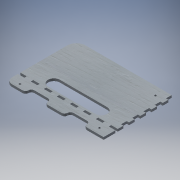
# Autodesk Inventor part: LatoPy
Saved by Autodesk Inventor 2018.3 (Build 223284000, 284)
## iProperties
Created: 2019-03-05
Part Number: LatoPy
Material: Generico
Document SubType Name: Modeling
Designer: AlfyPc
Density: 1 g/cm^3
Appearance: Legno - Verniciato - Bianco
Author: AlfyPc
Autodesk Inventor part; units mm, degrees
(part 1 of 3)
ref_plane "YZ Plane" through (0, 0, 0) normal (1, 0, 0) x (0, 1, 0)
ref_plane "XZ Plane" through (0, 0, 0) normal (0, 1, 0) x (-1, 0, 0)
ref_plane "XY Plane" through (0, 0, 0) normal (0, 0, 1) x (1, 0, 0)
sketch "Schizzo1" plane through (0, 0, 0) normal (0, 0, 1) x (1, 0, 0)
  line L0 (4, 17) -> (0, 17) construction
  line L1 (0, 17) -> (0, 95) construction
  line L2 (0, 95) -> (4, 95) construction
  line L3 (4, 95) -> (4, 17) construction
  line L4 (4, -4) -> (4, -24) construction
  line L5 (4, -24) -> (0, -24) construction
  line L6 (0, -24) -> (0, -4) construction
  line L7 (0, 0) -> (0, 11) construction
  line L8 (0, 11) -> (4, 11) construction
  line L9 (4, 11) -> (4, 0) construction
  line L10 (-161, -24) -> (-161, 95)
  line L11 (-161, 95) -> (4, 95)
  line L12 (4, 95) -> (4, -24)
  line L13 (-133, -24) -> (-161, -24)
  arc A0 (-133, -24) -> (-128, -19) centre (-133, -19) ccw
  arc A1 (-123, -14) -> (-128, -19) centre (-123, -19) ccw
  line L14 (-100, -14) -> (-123, -14)
  arc A2 (-95, -19) -> (-100, -14) centre (-100, -19) ccw
  arc A3 (-95, -19) -> (-90, -24) centre (-90, -19) ccw
  line L15 (-67, -24) -> (-90, -24)
  arc A4 (-67, -24) -> (-62, -19) centre (-67, -19) ccw
  arc A5 (-57, -14) -> (-62, -19) centre (-57, -19) ccw
  line L16 (-34, -14) -> (-57, -14)
  arc A6 (-29, -19) -> (-34, -14) centre (-34, -19) ccw
  arc A7 (-29, -19) -> (-24, -24) centre (-24, -19) ccw
  line L17 (4, -24) -> (-24, -24)
  line L18 (-117, 13) -> (-37, 13) construction
  line L19 (-117, 3) -> (-37, 3)
  line L20 (-37, 23) -> (-117, 23)
  arc A8 (-117, 23) -> (-117, 3) centre (-117, 13) ccw
  arc A9 (-37, 3) -> (-37, 23) centre (-37, 13) ccw
  line L21 (-161, -4) -> (-150, -4) projected
  line L22 (-150, 0) -> (-150, -4) projected
  line L23 (-139, -4) -> (-128, -4) projected
  line L24 (-128, 0) -> (-128, -4) projected
  line L25 (-139, 0) -> (-128, 0) projected
  line L26 (-139, 0) -> (-139, -4) projected
  line L27 (-117, -4) -> (-106, -4) projected
  line L28 (-106, 0) -> (-106, -4) projected
  line L29 (-117, 0) -> (-106, 0) projected
  line L30 (-117, 0) -> (-117, -4) projected
  line L31 (-95, -4) -> (-84, -4) projected
  line L32 (-84, 0) -> (-84, -4) projected
  line L33 (-95, 0) -> (-84, 0) projected
  line L34 (-95, 0) -> (-95, -4) projected
  line L35 (-73, -4) -> (-62, -4) projected
  line L36 (-62, 0) -> (-62, -4) projected
  line L37 (-73, 0) -> (-62, 0) projected
  line L38 (-73, 0) -> (-73, -4) projected
  line L39 (-51, -4) -> (-40, -4) projected
  line L40 (-40, 0) -> (-40, -4) projected
  line L41 (-51, 0) -> (-40, 0) projected
  line L42 (-51, 0) -> (-51, -4) projected
  line L43 (-29, -4) -> (-18, -4) projected
  line L44 (-18, 0) -> (-18, -4) projected
  line L45 (-29, 0) -> (-18, 0) projected
  line L46 (-29, 0) -> (-29, -4) projected
  line L47 (-7, -4) -> (4, -4) projected
  line L48 (4, 0) -> (4, -4) projected
  line L49 (-7, 0) -> (4, 0) projected
  line L50 (-7, 0) -> (-7, -4) projected
  line L51 (-161, 0) -> (-150, 0) projected
  line L52 (-161, 0) -> (-161, -4) projected
  point P0 (-77, 13)
  dimension "d0" = 80
  constraints: 44 end point, 20 point on circle, 10 centre point, 6 vertical, 4 horizontal, 4 tangent, 2 parallel, 1 midpoint, 10 other
  measures "d0" distance of L18.start L18.end
extrude "Estrusione1" add sketch "Schizzo1" along normal blind 4 contours L10 L21 L22 L51 L11 L12 L49 L50 L47 L17 A7 A6 L16 A5 A4 L15 A3 A2 L14 A1 A0 L13
sketch "Schizzo2" plane through (0, 0, 4) normal (0, 0, 1) x (1, 0, 0)
  line L0 (0, 76) -> (4, 76)
  line L1 (4, 76) -> (4, 66.5)
  line L2 (4, 66.5) -> (0, 66.5)
  line L3 (0, 66.5) -> (0, 76)
  line L4 (4, 85.5) -> (0, 85.5)
  line L5 (0, 85.5) -> (0, 95)
  line L6 (0, 95) -> (4, 95)
  line L7 (4, 95) -> (4, 85.5)
  line L8 (0, 38) -> (4, 38)
  line L9 (4, 38) -> (4, 28.5)
  line L10 (4, 28.5) -> (0, 28.5)
  line L11 (0, 28.5) -> (0, 38)
  line L12 (4, 47.5) -> (0, 47.5)
  line L13 (0, 47.5) -> (0, 57)
  line L14 (0, 57) -> (4, 57)
  line L15 (4, 57) -> (4, 47.5)
  line L16 (4, 9.5) -> (0, 9.5)
  line L17 (0, 9.5) -> (0, 19)
  line L18 (0, 19) -> (4, 19)
  line L19 (4, 19) -> (4, 9.5)
  point P0 (0, 0)
  constraints: 40 end point, 10 horizontal, 10 vertical, 20 other
extrude "Estrusione2" cut sketch "Schizzo2" against normal blind 4
fillet "Raccordo1" radius 15 1 edges at (-161, 95, 2)
fillet "Raccordo2" radius 10 1 edges at (-161, -24, 2)
sketch "Schizzo3" plane through (0, 0, 4) normal (0, 0, 1) x (1, 0, 0)
  line L0 (-146.15, 0) -> (-142.85, 0) projected
  line L1 (-14.15, 0) -> (-10.85, 0) projected
  line L2 (-144.5, 0) -> (-144.5, -17) construction
  circle A0 centre (-144.5, -17) radius 1.65
  line L3 (0, 79.1) -> (0, 82.4) construction
  line L4 (0, -15.65) -> (0, -12.35) construction
  line L5 (0, -14) -> (-13, -14) construction
  line L6 (0, 80.75) -> (-13, 80.75) construction
  circle A1 centre (-13, 80.75) radius 1.65
  circle A2 centre (-13, -14) radius 1.65
  point P0 (0, 0)
  dimension "d8" = 3.3
  dimension "d13" = 13
  dimension "d14" = 13
  dimension "d15" = 3.3
  dimension "d16" = 3.3
  dimension "d17" = 17
  constraints: 6 end point, 3 centre point, 3 coincident, 3 midpoint, 2 horizontal, 1 vertical
  measures "d8" diameter of A0
  measures "d13" distance of L5.start L5.end
  measures "d14" distance of L6.start L6.end
  measures "d15" diameter of A1
  measures "d16" diameter of A2
  measures "d17" distance of L2.start L2.end
extrude "Estrusione3" cut sketch "Schizzo3" against normal blind 4
sketch "Schizzo4" plane through (0, 0, 0) normal (0, 0, -1) x (-1, 0, 0)
  line L0 (22.8203, 78.8425) -> (60.2555, 78.8425)
  line L1 (60.2555, 78.8425) -> (60.2555, 30)
  line L2 (60.2555, 30) -> (22.8203, 30)
  line L3 (22.8203, 30) -> (22.8203, 78.8425)
  line L4 (68.3569, 29.9673) -> (68.3569, 80.7398) construction
  line L5 (68.3569, 80.7398) -> (122.609, 80.7398) construction
  line L6 (122.609, 80.7398) -> (122.609, 29.9673) construction
  line L7 (122.609, 29.9673) -> (68.3569, 29.9673) construction
  spline S0 degree 2 poles (71.5343, 79.079) (71.5343, 78.615) (71.1438, 77.902) (70.4223, 77.5144) (69.9498, 77.5144) knots 0 0 0 1 2 3 3 3
  line L8 (69.9498, 77.5144) -> (68.6568, 77.5144)
  line L9 (68.6568, 77.5144) -> (68.6568, 80.5644)
  line L10 (68.6568, 80.5644) -> (69.9215, 80.5644)
  spline S1 degree 2 poles (69.9215, 80.5644) (71.5343, 80.5644) (71.5343, 79.079) knots 0 0 0 1 1 1
  spline S2 degree 2 poles (70.5581, 79.0705) (70.5581, 79.2912) (70.3771, 79.6505) (70.0404, 79.8457) (69.814, 79.8457) knots 0 0 0 1 2 3 3 3
  line L11 (69.814, 79.8457) -> (69.5764, 79.8457)
  line L12 (69.5764, 79.8457) -> (69.5764, 78.233)
  line L13 (69.5764, 78.233) -> (69.8338, 78.233)
  spline S3 degree 2 poles (69.8338, 78.233) (70.1649, 78.233) (70.5581, 78.6857) (70.5581, 79.0705) knots 0 0 0 1 2 2 2
  spline S4 degree 2 poles (72.6632, 78.3462) (72.6858, 78.2047) (72.9631, 78.0463) (73.1894, 78.0463) knots 0 0 0 1 2 2 2
  spline S5 degree 2 poles (73.1894, 78.0463) (73.5063, 78.0463) (73.7892, 78.1679) knots 0 0 0 1 1 1
  line L14 (73.7892, 78.1679) -> (73.7892, 77.5936)
  spline S6 degree 2 poles (73.7892, 77.5936) (73.461, 77.4606) (72.9885, 77.4606) knots 0 0 0 1 1 1
  spline S7 degree 2 poles (72.9885, 77.4606) (72.4198, 77.4606) (71.7861, 78.0435) (71.7861, 78.5556) knots 0 0 0 1 2 2 2
  spline S8 degree 2 poles (71.7861, 78.5556) (71.7861, 78.9064) (72.0633, 79.4411) (72.6094, 79.7467) (72.9404, 79.7467) knots 0 0 0 1 2 3 3 3
  spline S9 degree 2 poles (72.9404, 79.7467) (73.2771, 79.7467) (73.7581, 79.4836) (74.0071, 79.0054) (74.0071, 78.6857) knots 0 0 0 1 2 3 3 3
  line L15 (74.0071, 78.6857) -> (74.0071, 78.3462)
  line L16 (74.0071, 78.3462) -> (72.6632, 78.3462)
  spline S10 degree 2 poles (73.2064, 78.8215) (73.2064, 79.1978) (72.9376, 79.1978) knots 0 0 0 1 1 1
  spline S11 degree 2 poles (72.9376, 79.1978) (72.8244, 79.1978) (72.6716, 78.9913) (72.6575, 78.8215) knots 0 0 0 1 2 2 2
  line L17 (72.6575, 78.8215) -> (73.2064, 78.8215)
  line L18 (75.9055, 77.5144) -> (74.8304, 77.5144)
  line L19 (74.8304, 77.5144) -> (74.1033, 79.6929)
  line L20 (74.1033, 79.6929) -> (75.0483, 79.6929)
  line L21 (75.0483, 79.6929) -> (75.3142, 78.5046)
  spline S12 degree 2 poles (75.3142, 78.5046) (75.3765, 78.216) (75.385, 78.0718) knots 0 0 0 1 1 1
  line L22 (75.385, 78.0718) -> (75.3963, 78.0718)
  spline S13 degree 2 poles (75.3963, 78.0718) (75.4019, 78.1142) (75.4161, 78.2047) (75.7245, 79.6929) knots 0 0 0 1 2 2 2
  line L23 (75.7245, 79.6929) -> (76.6638, 79.6929)
  line L24 (76.6638, 79.6929) -> (75.9055, 77.5144)
  spline S14 degree 2 poles (77.6625, 78.3462) (77.6852, 78.2047) (77.9625, 78.0463) (78.1888, 78.0463) knots 0 0 0 1 2 2 2
  spline S15 degree 2 poles (78.1888, 78.0463) (78.5057, 78.0463) (78.7886, 78.1679) knots 0 0 0 1 1 1
  line L25 (78.7886, 78.1679) -> (78.7886, 77.5936)
  spline S16 degree 2 poles (78.7886, 77.5936) (78.4604, 77.4606) (77.9879, 77.4606) knots 0 0 0 1 1 1
  spline S17 degree 2 poles (77.9879, 77.4606) (77.4192, 77.4606) (76.7855, 78.0435) (76.7855, 78.5556) knots 0 0 0 1 2 2 2
  spline S18 degree 2 poles (76.7855, 78.5556) (76.7855, 78.9064) (77.0627, 79.4411) (77.6088, 79.7467) (77.9398, 79.7467) knots 0 0 0 1 2 3 3 3
  spline S19 degree 2 poles (77.9398, 79.7467) (78.2765, 79.7467) (78.7575, 79.4836) (79.0065, 79.0054) (79.0065, 78.6857) knots 0 0 0 1 2 3 3 3
  line L26 (79.0065, 78.6857) -> (79.0065, 78.3462)
  line L27 (79.0065, 78.3462) -> (77.6625, 78.3462)
  spline S20 degree 2 poles (78.2058, 78.8215) (78.2058, 79.1978) (77.937, 79.1978) knots 0 0 0 1 1 1
  spline S21 degree 2 poles (77.937, 79.1978) (77.8238, 79.1978) (77.671, 78.9913) (77.6569, 78.8215) knots 0 0 0 1 2 2 2
  line L28 (77.6569, 78.8215) -> (78.2058, 78.8215)
  line L29 (79.3205, 77.5144) -> (79.3205, 80.7398)
  line L30 (79.3205, 80.7398) -> (80.2259, 80.7398)
  line L31 (80.2259, 80.7398) -> (80.2259, 77.5144)
  line L32 (80.2259, 77.5144) -> (79.3205, 77.5144)
  spline S22 degree 2 poles (83.0835, 78.6433) (83.0835, 78.0916) (82.4186, 77.4606) (81.8216, 77.4606) knots 0 0 0 1 2 2 2
  spline S23 degree 2 poles (81.8216, 77.4606) (81.2275, 77.4606) (80.5654, 78.0746) (80.5654, 78.6178) knots 0 0 0 1 2 2 2
  spline S24 degree 2 poles (80.5654, 78.6178) (80.5654, 78.963) (80.8766, 79.4751) (81.451, 79.7467) (81.8245, 79.7467) knots 0 0 0 1 2 3 3 3
  spline S25 degree 2 poles (81.8245, 79.7467) (82.2121, 79.7467) (82.7808, 79.4609) (83.0835, 78.9545) (83.0835, 78.6433) knots 0 0 0 1 2 3 3 3
  spline S26 degree 2 poles (82.164, 78.6376) (82.164, 79.0818) (81.8245, 79.0818) knots 0 0 0 1 1 1
  spline S27 degree 2 poles (81.8245, 79.0818) (81.485, 79.0818) (81.485, 78.6178) knots 0 0 0 1 1 1
  spline S28 degree 2 poles (81.485, 78.6178) (81.485, 78.1255) (81.8301, 78.1255) knots 0 0 0 1 1 1
  spline S29 degree 2 poles (81.8301, 78.1255) (82.164, 78.1255) (82.164, 78.6376) knots 0 0 0 1 1 1
  spline S30 degree 2 poles (85.8789, 78.6687) (85.8789, 78.3122) (85.6356, 77.7634) (85.1942, 77.4606) (84.9169, 77.4606) knots 0 0 0 1 2 3 3 3
  spline S31 degree 2 poles (84.9169, 77.4606) (84.535, 77.4606) (84.3369, 77.7407) knots 0 0 0 1 1 1
  line L33 (84.3369, 77.7407) -> (84.3284, 77.7407)
  line L34 (84.3284, 77.7407) -> (84.3284, 76.5128)
  line L35 (84.3284, 76.5128) -> (83.423, 76.5128)
  line L36 (83.423, 76.5128) -> (83.423, 79.6929)
  line L37 (83.423, 79.6929) -> (84.3284, 79.6929)
  line L38 (84.3284, 79.6929) -> (84.3284, 79.3959)
  line L39 (84.3284, 79.3959) -> (84.3369, 79.3959)
  spline S32 degree 2 poles (84.3369, 79.3959) (84.4444, 79.56) (84.7896, 79.7467) (85.0103, 79.7467) knots 0 0 0 1 2 2 2
  spline S33 degree 2 poles (85.0103, 79.7467) (85.429, 79.7467) (85.8789, 79.1837) (85.8789, 78.6687) knots 0 0 0 1 2 2 2
  spline S34 degree 2 poles (84.9593, 78.6433) (84.9593, 78.847) (84.8009, 79.0818) (84.634, 79.0818) knots 0 0 0 1 2 2 2
  spline S35 degree 2 poles (84.634, 79.0818) (84.4897, 79.0818) (84.3114, 78.8357) (84.3114, 78.6206) knots 0 0 0 1 2 2 2
  line L40 (84.3114, 78.6206) -> (84.3114, 78.5782)
  spline S36 degree 2 poles (84.3114, 78.5782) (84.3114, 78.3717) (84.4642, 78.1255) (84.617, 78.1255) knots 0 0 0 1 2 2 2
  spline S37 degree 2 poles (84.617, 78.1255) (84.7811, 78.1255) (84.9593, 78.3943) (84.9593, 78.6433) knots 0 0 0 1 2 2 2
  spline S38 degree 2 poles (87.0021, 78.3462) (87.0247, 78.2047) (87.302, 78.0463) (87.5284, 78.0463) knots 0 0 0 1 2 2 2
  spline S39 degree 2 poles (87.5284, 78.0463) (87.8452, 78.0463) (88.1282, 78.1679) knots 0 0 0 1 1 1
  line L41 (88.1282, 78.1679) -> (88.1282, 77.5936)
  spline S40 degree 2 poles (88.1282, 77.5936) (87.8, 77.4606) (87.3275, 77.4606) knots 0 0 0 1 1 1
  spline S41 degree 2 poles (87.3275, 77.4606) (86.7588, 77.4606) (86.125, 78.0435) (86.125, 78.5556) knots 0 0 0 1 2 2 2
  spline S42 degree 2 poles (86.125, 78.5556) (86.125, 78.9064) (86.4023, 79.4411) (86.9484, 79.7467) (87.2794, 79.7467) knots 0 0 0 1 2 3 3 3
  spline S43 degree 2 poles (87.2794, 79.7467) (87.6161, 79.7467) (88.0971, 79.4836) (88.346, 79.0054) (88.346, 78.6857) knots 0 0 0 1 2 3 3 3
  line L42 (88.346, 78.6857) -> (88.346, 78.3462)
  line L43 (88.346, 78.3462) -> (87.0021, 78.3462)
  spline S44 degree 2 poles (87.5453, 78.8215) (87.5453, 79.1978) (87.2766, 79.1978) knots 0 0 0 1 1 1
  spline S45 degree 2 poles (87.2766, 79.1978) (87.1634, 79.1978) (87.0106, 78.9913) (86.9965, 78.8215) knots 0 0 0 1 2 2 2
  line L44 (86.9965, 78.8215) -> (87.5453, 78.8215)
  line L45 (90.1144, 77.5144) -> (90.1144, 77.769)
  line L46 (90.1144, 77.769) -> (90.1059, 77.769)
  spline S46 degree 2 poles (90.1059, 77.769) (89.9984, 77.6247) (89.6475, 77.4606) (89.4778, 77.4606) knots 0 0 0 1 2 2 2
  spline S47 degree 2 poles (89.4778, 77.4606) (89.2005, 77.4606) (88.7733, 77.7351) (88.5639, 78.2302) (88.5639, 78.5641) knots 0 0 0 1 2 3 3 3
  spline S48 degree 2 poles (88.5639, 78.5641) (88.5639, 78.9121) (88.8157, 79.4496) (89.2712, 79.7467) (89.5542, 79.7467) knots 0 0 0 1 2 3 3 3
  spline S49 degree 2 poles (89.5542, 79.7467) (89.6871, 79.7467) (89.9135, 79.6703) (90.0832, 79.5402) (90.1059, 79.4751) knots 0 0 0 1 2 3 3 3
  line L47 (90.1059, 79.4751) -> (90.1144, 79.4751)
  line L48 (90.1144, 79.4751) -> (90.1144, 80.7398)
  line L49 (90.1144, 80.7398) -> (91.0197, 80.7398)
  line L50 (91.0197, 80.7398) -> (91.0197, 77.5144)
  line L51 (91.0197, 77.5144) -> (90.1144, 77.5144)
  spline S50 degree 2 poles (90.1342, 78.6687) (90.1342, 78.864) (89.9616, 79.0818) (89.8144, 79.0818) knots 0 0 0 1 2 2 2
  spline S51 degree 2 poles (89.8144, 79.0818) (89.6673, 79.0818) (89.4834, 78.813) (89.4834, 78.5867) knots 0 0 0 1 2 2 2
  spline S52 degree 2 poles (89.4834, 78.5867) (89.4834, 78.1255) (89.8031, 78.1255) knots 0 0 0 1 1 1
  spline S53 degree 2 poles (89.8031, 78.1255) (89.9531, 78.1255) (90.1342, 78.3745) (90.1342, 78.6122) knots 0 0 0 1 2 2 2
  line L52 (90.1342, 78.6122) -> (90.1342, 78.6687)
  spline S54 degree 2 poles (95.1251, 78.6687) (95.1251, 78.3122) (94.8902, 77.7605) (94.4545, 77.4606) (94.1801, 77.4606) knots 0 0 0 1 2 3 3 3
  spline S55 degree 2 poles (94.1801, 77.4606) (93.9707, 77.4606) (93.6708, 77.6162) (93.5831, 77.7407) knots 0 0 0 1 2 2 2
  line L53 (93.5831, 77.7407) -> (93.5746, 77.7407)
  line L54 (93.5746, 77.7407) -> (93.5746, 77.5144)
  line L55 (93.5746, 77.5144) -> (92.6692, 77.5144)
  line L56 (92.6692, 77.5144) -> (92.6692, 80.7398)
  line L57 (92.6692, 80.7398) -> (93.5746, 80.7398)
  line L58 (93.5746, 80.7398) -> (93.5746, 79.3987)
  line L59 (93.5746, 79.3987) -> (93.5831, 79.3987)
  spline S56 degree 2 poles (93.5831, 79.3987) (93.6906, 79.56) (94.0528, 79.7467) (94.2734, 79.7467) knots 0 0 0 1 2 2 2
  spline S57 degree 2 poles (94.2734, 79.7467) (94.6837, 79.7467) (95.1251, 79.1978) (95.1251, 78.6687) knots 0 0 0 1 2 2 2
  spline S58 degree 2 poles (94.2055, 78.6433) (94.2055, 78.8611) (94.0386, 79.0818) (93.8802, 79.0818) knots 0 0 0 1 2 2 2
  spline S59 degree 2 poles (93.8802, 79.0818) (93.7415, 79.0818) (93.5576, 78.8498) (93.5576, 78.6659) knots 0 0 0 1 2 2 2
  line L60 (93.5576, 78.6659) -> (93.5576, 78.5329)
  spline S60 degree 2 poles (93.5576, 78.5329) (93.5576, 78.3462) (93.7246, 78.1255) (93.8632, 78.1255) knots 0 0 0 1 2 2 2
  spline S61 degree 2 poles (93.8632, 78.1255) (94.0273, 78.1255) (94.2055, 78.3943) (94.2055, 78.6433) knots 0 0 0 1 2 2 2
  spline S62 degree 2 poles (95.889, 76.4902) (95.7617, 76.4902) (95.4702, 76.5354) (95.3542, 76.5779) knots 0 0 0 1 2 2 2
  line L61 (95.3542, 76.5779) -> (95.3542, 77.2597)
  spline S63 degree 2 poles (95.3542, 77.2597) (95.408, 77.2201) (95.6174, 77.1522) (95.7107, 77.1522) knots 0 0 0 1 2 2 2
  spline S64 degree 2 poles (95.7107, 77.1522) (95.9654, 77.1522) (96.0474, 77.3531) knots 0 0 0 1 1 1
  line L62 (96.0474, 77.3531) -> (96.1182, 77.5229)
  line L63 (96.1182, 77.5229) -> (95.2071, 79.6929)
  line L64 (95.2071, 79.6929) -> (96.2087, 79.6929)
  line L65 (96.2087, 79.6929) -> (96.4718, 78.6433)
  spline S65 degree 2 poles (96.4718, 78.6433) (96.5482, 78.349) (96.5567, 78.2472) knots 0 0 0 1 1 1
  line L66 (96.5567, 78.2472) -> (96.5652, 78.2472)
  spline S66 degree 2 poles (96.5652, 78.2472) (96.5709, 78.2953) (96.5935, 78.4084) (96.9132, 79.6929) knots 0 0 0 1 2 2 2
  line L67 (96.9132, 79.6929) -> (97.7931, 79.6929)
  line L68 (97.7931, 79.6929) -> (96.9924, 77.4521)
  spline S67 degree 2 poles (96.9924, 77.4521) (96.8113, 76.9372) (96.2766, 76.4902) (95.889, 76.4902) knots 0 0 0 1 2 2 2
  spline S68 degree 2 poles (98.9531, 77.8935) (98.9531, 77.6983) (98.6815, 77.4606) (98.441, 77.4606) knots 0 0 0 1 2 2 2
  spline S69 degree 2 poles (98.441, 77.4606) (98.2203, 77.4606) (97.9431, 77.7096) (97.9431, 77.8935) knots 0 0 0 1 2 2 2
  spline S70 degree 2 poles (97.9431, 77.8935) (97.9431, 78.0802) (98.2175, 78.3122) (98.4495, 78.3122) knots 0 0 0 1 2 2 2
  spline S71 degree 2 poles (98.4495, 78.3122) (98.6759, 78.3122) (98.9531, 78.0802) (98.9531, 77.8935) knots 0 0 0 1 2 2 2
  spline S72 degree 2 poles (98.9531, 79.2742) (98.9531, 79.079) (98.6787, 78.8442) (98.441, 78.8442) knots 0 0 0 1 2 2 2
  spline S73 degree 2 poles (98.441, 78.8442) (98.2232, 78.8442) (97.9431, 79.0903) (97.9431, 79.2742) knots 0 0 0 1 2 2 2
  spline S74 degree 2 poles (97.9431, 79.2742) (97.9431, 79.4609) (98.2175, 79.6929) (98.4495, 79.6929) knots 0 0 0 1 2 2 2
  spline S75 degree 2 poles (98.4495, 79.6929) (98.6759, 79.6929) (98.9531, 79.4609) (98.9531, 79.2742) knots 0 0 0 1 2 2 2
  spline S76 degree 2 poles (69.93, 72.6161) (69.93, 72.452) (69.7603, 72.1606) (69.4689, 71.9936) (69.3076, 71.9936) knots 0 0 0 1 2 3 3 3
  spline S77 degree 2 poles (69.3076, 71.9936) (69.0558, 71.9936) (68.6936, 72.3558) (68.6936, 72.6161) knots 0 0 0 1 2 2 2
  spline S78 degree 2 poles (68.6936, 72.6161) (68.6936, 72.8679) (69.0501, 73.23) (69.3076, 73.23) knots 0 0 0 1 2 2 2
  spline S79 degree 2 poles (69.3076, 73.23) (69.5707, 73.23) (69.93, 72.8622) (69.93, 72.6161) knots 0 0 0 1 2 2 2
  line L69 (79.7195, 71.5777) -> (79.5865, 72.1379)
  line L70 (79.5865, 72.1379) -> (78.6754, 72.1379)
  line L71 (78.6754, 72.1379) -> (78.5311, 71.5777)
  line L72 (78.5311, 71.5777) -> (77.5381, 71.5777)
  line L73 (77.5381, 71.5777) -> (78.5877, 74.6277)
  line L74 (78.5877, 74.6277) -> (79.7279, 74.6277)
  line L75 (79.7279, 74.6277) -> (80.7182, 71.5777)
  line L76 (80.7182, 71.5777) -> (79.7195, 71.5777)
  line L77 (79.1423, 73.9628) -> (79.1225, 73.9628)
  spline S80 degree 2 poles (79.1225, 73.9628) (79.1168, 73.9119) (79.0659, 73.6771) (78.8339, 72.7915) knots 0 0 0 1 2 2 2
  line L78 (78.8339, 72.7915) -> (79.4167, 72.7915)
  line L79 (79.4167, 72.7915) -> (79.2045, 73.6205)
  spline S81 degree 2 poles (79.2045, 73.6205) (79.1593, 73.8044) (79.1423, 73.9628) knots 0 0 0 1 1 1
  line L80 (80.9926, 71.5777) -> (80.9926, 74.8031)
  line L81 (80.9926, 74.8031) -> (81.898, 74.8031)
  line L82 (81.898, 74.8031) -> (81.898, 71.5777)
  line L83 (81.898, 71.5777) -> (80.9926, 71.5777)
  spline S82 degree 2 poles (84.0115, 74.1439) (83.8701, 74.192) (83.7512, 74.192) knots 0 0 0 1 1 1
  spline S83 degree 2 poles (83.7512, 74.192) (83.5984, 74.192) (83.4542, 74.0364) (83.4542, 73.9062) knots 0 0 0 1 2 2 2
  line L84 (83.4542, 73.9062) -> (83.4542, 73.7563)
  line L85 (83.4542, 73.7563) -> (83.9578, 73.7563)
  line L86 (83.9578, 73.7563) -> (83.9578, 73.1282)
  line L87 (83.9578, 73.1282) -> (83.4542, 73.1282)
  line L88 (83.4542, 73.1282) -> (83.4542, 71.5777)
  line L89 (83.4542, 71.5777) -> (82.5488, 71.5777)
  line L90 (82.5488, 71.5777) -> (82.5488, 73.1282)
  line L91 (82.5488, 73.1282) -> (82.1838, 73.1282)
  line L92 (82.1838, 73.1282) -> (82.1838, 73.7563)
  line L93 (82.1838, 73.7563) -> (82.5488, 73.7563)
  line L94 (82.5488, 73.7563) -> (82.5488, 73.9572)
  spline S84 degree 2 poles (82.5488, 73.9572) (82.5488, 74.2231) (82.7949, 74.6277) (83.2646, 74.8541) (83.6013, 74.8541) knots 0 0 0 1 2 3 3 3
  spline S85 degree 2 poles (83.6013, 74.8541) (83.8446, 74.8541) (84.0115, 74.806) knots 0 0 0 1 1 1
  line L95 (84.0115, 74.806) -> (84.0115, 74.1439)
  line L96 (85.4205, 71.5777) -> (85.4205, 71.9087)
  line L97 (85.4205, 71.9087) -> (85.412, 71.9087)
  spline S86 degree 2 poles (85.412, 71.9087) (85.1942, 71.524) (84.7471, 71.524) knots 0 0 0 1 1 1
  spline S87 degree 2 poles (84.7471, 71.524) (84.4388, 71.524) (84.0907, 71.8889) (84.0907, 72.1973) knots 0 0 0 1 2 2 2
  spline S88 degree 2 poles (84.0907, 72.1973) (84.0907, 72.8396) (84.8801, 72.9414) knots 0 0 0 1 1 1
  line L98 (84.8801, 72.9414) -> (85.4205, 73.0122)
  spline S89 degree 2 poles (85.4205, 73.0122) (85.4205, 73.1197) (85.2281, 73.2555) (85.0669, 73.2555) knots 0 0 0 1 2 2 2
  spline S90 degree 2 poles (85.0669, 73.2555) (84.7019, 73.2555) (84.2945, 73.0461) knots 0 0 0 1 1 1
  line L99 (84.2945, 73.0461) -> (84.2945, 73.6346)
  spline S91 degree 2 poles (84.2945, 73.6346) (84.4699, 73.711) (85.0046, 73.81) (85.1942, 73.81) knots 0 0 0 1 2 2 2
  spline S92 degree 2 poles (85.1942, 73.81) (85.7487, 73.81) (86.2495, 73.3347) (86.2495, 72.7802) knots 0 0 0 1 2 2 2
  line L100 (86.2495, 72.7802) -> (86.2495, 71.5777)
  line L101 (86.2495, 71.5777) -> (85.4205, 71.5777)
  spline S93 degree 2 poles (84.883, 72.319) (84.883, 72.2313) (84.9961, 72.1153) (85.1008, 72.1153) knots 0 0 0 1 2 2 2
  spline S94 degree 2 poles (85.1008, 72.1153) (85.2423, 72.1153) (85.4205, 72.3275) (85.4205, 72.4944) knots 0 0 0 1 2 2 2
  line L102 (85.4205, 72.4944) -> (85.4205, 72.5765)
  line L103 (85.4205, 72.5765) -> (85.1121, 72.534)
  spline S95 degree 2 poles (85.1121, 72.534) (84.883, 72.4944) (84.883, 72.319) knots 0 0 0 1 1 1
  line L104 (88.0688, 71.5777) -> (88.0688, 72.766)
  spline S96 degree 2 poles (88.0688, 72.766) (88.0688, 72.9697) (87.9471, 73.1452) (87.8113, 73.1452) knots 0 0 0 1 2 2 2
  spline S97 degree 2 poles (87.8113, 73.1452) (87.6953, 73.1452) (87.5623, 72.9612) (87.5623, 72.8198) knots 0 0 0 1 2 2 2
  line L105 (87.5623, 72.8198) -> (87.5623, 71.5777)
  line L106 (87.5623, 71.5777) -> (86.6569, 71.5777)
  line L107 (86.6569, 71.5777) -> (86.6569, 73.7563)
  line L108 (86.6569, 73.7563) -> (87.5623, 73.7563)
  line L109 (87.5623, 73.7563) -> (87.5623, 73.4168)
  line L110 (87.5623, 73.4168) -> (87.5708, 73.4168)
  spline S98 degree 2 poles (87.5708, 73.4168) (87.6783, 73.6035) (88.0461, 73.81) (88.2612, 73.81) knots 0 0 0 1 2 2 2
  spline S99 degree 2 poles (88.2612, 73.81) (88.9741, 73.81) (88.9741, 72.9075) knots 0 0 0 1 1 1
  line L111 (88.9741, 72.9075) -> (88.9741, 71.5777)
  line L112 (88.9741, 71.5777) -> (88.0688, 71.5777)
  spline S100 degree 2 poles (91.8063, 72.7066) (91.8063, 72.1549) (91.1414, 71.524) (90.5444, 71.524) knots 0 0 0 1 2 2 2
  spline S101 degree 2 poles (90.5444, 71.524) (89.9503, 71.524) (89.2882, 72.1379) (89.2882, 72.6811) knots 0 0 0 1 2 2 2
  spline S102 degree 2 poles (89.2882, 72.6811) (89.2882, 73.0263) (89.5994, 73.5384) (90.1738, 73.81) (90.5472, 73.81) knots 0 0 0 1 2 3 3 3
  spline S103 degree 2 poles (90.5472, 73.81) (90.9349, 73.81) (91.5035, 73.5243) (91.8063, 73.0178) (91.8063, 72.7066) knots 0 0 0 1 2 3 3 3
  spline S104 degree 2 poles (90.8868, 72.701) (90.8868, 73.1452) (90.5472, 73.1452) knots 0 0 0 1 1 1
  spline S105 degree 2 poles (90.5472, 73.1452) (90.2077, 73.1452) (90.2077, 72.6811) knots 0 0 0 1 1 1
  spline S106 degree 2 poles (90.2077, 72.6811) (90.2077, 72.1888) (90.5529, 72.1888) knots 0 0 0 1 1 1
  spline S107 degree 2 poles (90.5529, 72.1888) (90.8868, 72.1888) (90.8868, 72.701) knots 0 0 0 1 1 1
  line L113 (93.4388, 71.5777) -> (93.4388, 74.6277)
  line L114 (93.4388, 74.6277) -> (95.3373, 74.6277)
  line L115 (95.3373, 74.6277) -> (95.3373, 73.9091)
  line L116 (95.3373, 73.9091) -> (94.3583, 73.9091)
  line L117 (94.3583, 73.9091) -> (94.3583, 73.4649)
  line L118 (94.3583, 73.4649) -> (95.2779, 73.4649)
  line L119 (95.2779, 73.4649) -> (95.2779, 72.7462)
  line L120 (95.2779, 72.7462) -> (94.3583, 72.7462)
  line L121 (94.3583, 72.7462) -> (94.3583, 72.2964)
  line L122 (94.3583, 72.2964) -> (95.408, 72.2964)
  line L123 (95.408, 72.2964) -> (95.408, 71.5777)
  line L124 (95.408, 71.5777) -> (93.4388, 71.5777)
  line L125 (98.5853, 71.5777) -> (98.5853, 72.8339)
  spline S108 degree 2 poles (98.5853, 72.8339) (98.5853, 72.9895) (98.4721, 73.1452) (98.3448, 73.1452) knots 0 0 0 1 2 2 2
  spline S109 degree 2 poles (98.3448, 73.1452) (98.2203, 73.1452) (98.0789, 72.9556) (98.0789, 72.7887) knots 0 0 0 1 2 2 2
  line L126 (98.0789, 72.7887) -> (98.0789, 71.5777)
  line L127 (98.0789, 71.5777) -> (97.1735, 71.5777)
  line L128 (97.1735, 71.5777) -> (97.1735, 72.8113)
  spline S110 degree 2 poles (97.1735, 72.8113) (97.1735, 73.1452) (96.9471, 73.1452) knots 0 0 0 1 1 1
  spline S111 degree 2 poles (96.9471, 73.1452) (96.8085, 73.1452) (96.667, 72.9528) (96.667, 72.7717) knots 0 0 0 1 2 2 2
  line L129 (96.667, 72.7717) -> (96.667, 71.5777)
  line L130 (96.667, 71.5777) -> (95.7617, 71.5777)
  line L131 (95.7617, 71.5777) -> (95.7617, 73.7563)
  line L132 (95.7617, 73.7563) -> (96.667, 73.7563)
  line L133 (96.667, 73.7563) -> (96.667, 73.4111)
  line L134 (96.667, 73.4111) -> (96.6755, 73.4111)
  spline S112 degree 2 poles (96.6755, 73.4111) (96.7265, 73.5016) (96.95, 73.694) (97.2301, 73.81) (97.3942, 73.81) knots 0 0 0 1 2 3 3 3
  spline S113 degree 2 poles (97.3942, 73.81) (97.6262, 73.81) (97.9431, 73.6261) (98.0478, 73.4281) knots 0 0 0 1 2 2 2
  spline S114 degree 2 poles (98.0478, 73.4281) (98.1638, 73.612) (98.5485, 73.81) (98.7805, 73.81) knots 0 0 0 1 2 2 2
  spline S115 degree 2 poles (98.7805, 73.81) (99.1257, 73.81) (99.4907, 73.363) (99.4907, 72.9414) knots 0 0 0 1 2 2 2
  line L135 (99.4907, 72.9414) -> (99.4907, 71.5777)
  line L136 (99.4907, 71.5777) -> (98.5853, 71.5777)
  line L137 (101.1091, 71.5777) -> (101.1091, 71.9087)
  line L138 (101.1091, 71.9087) -> (101.1006, 71.9087)
  spline S116 degree 2 poles (101.1006, 71.9087) (100.8827, 71.524) (100.4357, 71.524) knots 0 0 0 1 1 1
  spline S117 degree 2 poles (100.4357, 71.524) (100.1273, 71.524) (99.7793, 71.8889) (99.7793, 72.1973) knots 0 0 0 1 2 2 2
  spline S118 degree 2 poles (99.7793, 72.1973) (99.7793, 72.8396) (100.5687, 72.9414) knots 0 0 0 1 1 1
  line L139 (100.5687, 72.9414) -> (101.1091, 73.0122)
  spline S119 degree 2 poles (101.1091, 73.0122) (101.1091, 73.1197) (100.9167, 73.2555) (100.7554, 73.2555) knots 0 0 0 1 2 2 2
  spline S120 degree 2 poles (100.7554, 73.2555) (100.3904, 73.2555) (99.983, 73.0461) knots 0 0 0 1 1 1
  line L140 (99.983, 73.0461) -> (99.983, 73.6346)
  spline S121 degree 2 poles (99.983, 73.6346) (100.1584, 73.711) (100.6932, 73.81) (100.8827, 73.81) knots 0 0 0 1 2 2 2
  spline S122 degree 2 poles (100.8827, 73.81) (101.4373, 73.81) (101.9381, 73.3347) (101.9381, 72.7802) knots 0 0 0 1 2 2 2
  line L141 (101.9381, 72.7802) -> (101.9381, 71.5777)
  line L142 (101.9381, 71.5777) -> (101.1091, 71.5777)
  spline S123 degree 2 poles (100.5715, 72.319) (100.5715, 72.2313) (100.6847, 72.1153) (100.7894, 72.1153) knots 0 0 0 1 2 2 2
  spline S124 degree 2 poles (100.7894, 72.1153) (100.9308, 72.1153) (101.1091, 72.3275) (101.1091, 72.4944) knots 0 0 0 1 2 2 2
  line L143 (101.1091, 72.4944) -> (101.1091, 72.5765)
  line L144 (101.1091, 72.5765) -> (100.8007, 72.534)
  spline S125 degree 2 poles (100.8007, 72.534) (100.5715, 72.4944) (100.5715, 72.319) knots 0 0 0 1 1 1
  line L145 (103.7573, 71.5777) -> (103.7573, 72.766)
  spline S126 degree 2 poles (103.7573, 72.766) (103.7573, 72.9697) (103.6356, 73.1452) (103.4998, 73.1452) knots 0 0 0 1 2 2 2
  spline S127 degree 2 poles (103.4998, 73.1452) (103.3838, 73.1452) (103.2509, 72.9612) (103.2509, 72.8198) knots 0 0 0 1 2 2 2
  line L146 (103.2509, 72.8198) -> (103.2509, 71.5777)
  line L147 (103.2509, 71.5777) -> (102.3455, 71.5777)
  line L148 (102.3455, 71.5777) -> (102.3455, 73.7563)
  line L149 (102.3455, 73.7563) -> (103.2509, 73.7563)
  line L150 (103.2509, 73.7563) -> (103.2509, 73.4168)
  line L151 (103.2509, 73.4168) -> (103.2593, 73.4168)
  spline S128 degree 2 poles (103.2593, 73.4168) (103.3669, 73.6035) (103.7347, 73.81) (103.9497, 73.81) knots 0 0 0 1 2 2 2
  spline S129 degree 2 poles (103.9497, 73.81) (104.6627, 73.81) (104.6627, 72.9075) knots 0 0 0 1 1 1
  line L152 (104.6627, 72.9075) -> (104.6627, 71.5777)
  line L153 (104.6627, 71.5777) -> (103.7573, 71.5777)
  line L154 (106.4593, 71.5777) -> (106.4593, 71.9144)
  line L155 (106.4593, 71.9144) -> (106.4508, 71.9144)
  spline S130 degree 2 poles (106.4508, 71.9144) (106.3376, 71.7588) (106.1566, 71.6145) (105.9302, 71.524) (105.7803, 71.524) knots 0 0 0 1 2 3 3 3
  spline S131 degree 2 poles (105.7803, 71.524) (105.4209, 71.524) (105.0475, 71.988) (105.0475, 72.4407) knots 0 0 0 1 2 2 2
  line L156 (105.0475, 72.4407) -> (105.0475, 73.7563)
  line L157 (105.0475, 73.7563) -> (105.9529, 73.7563)
  line L158 (105.9529, 73.7563) -> (105.9529, 72.5114)
  spline S132 degree 2 poles (105.9529, 72.5114) (105.9529, 72.1888) (106.1933, 72.1888) knots 0 0 0 1 1 1
  spline S133 degree 2 poles (106.1933, 72.1888) (106.3263, 72.1888) (106.4593, 72.3643) (106.4593, 72.5227) knots 0 0 0 1 2 2 2
  line L159 (106.4593, 72.5227) -> (106.4593, 73.7563)
  line L160 (106.4593, 73.7563) -> (107.3647, 73.7563)
  line L161 (107.3647, 73.7563) -> (107.3647, 71.5777)
  line L162 (107.3647, 71.5777) -> (106.4593, 71.5777)
  spline S134 degree 2 poles (108.5813, 72.4095) (108.6039, 72.2681) (108.8812, 72.1096) (109.1075, 72.1096) knots 0 0 0 1 2 2 2
  spline S135 degree 2 poles (109.1075, 72.1096) (109.4244, 72.1096) (109.7074, 72.2313) knots 0 0 0 1 1 1
  line L163 (109.7074, 72.2313) -> (109.7074, 71.6569)
  spline S136 degree 2 poles (109.7074, 71.6569) (109.3792, 71.524) (108.9067, 71.524) knots 0 0 0 1 1 1
  spline S137 degree 2 poles (108.9067, 71.524) (108.338, 71.524) (107.7042, 72.1068) (107.7042, 72.6189) knots 0 0 0 1 2 2 2
  spline S138 degree 2 poles (107.7042, 72.6189) (107.7042, 72.9697) (107.9815, 73.5045) (108.5275, 73.81) (108.8586, 73.81) knots 0 0 0 1 2 3 3 3
  spline S139 degree 2 poles (108.8586, 73.81) (109.1952, 73.81) (109.6762, 73.5469) (109.9252, 73.0688) (109.9252, 72.749) knots 0 0 0 1 2 3 3 3
  line L164 (109.9252, 72.749) -> (109.9252, 72.4095)
  line L165 (109.9252, 72.4095) -> (108.5813, 72.4095)
  spline S140 degree 2 poles (109.1245, 72.8849) (109.1245, 73.2612) (108.8557, 73.2612) knots 0 0 0 1 1 1
  spline S141 degree 2 poles (108.8557, 73.2612) (108.7426, 73.2612) (108.5898, 73.0546) (108.5756, 72.8849) knots 0 0 0 1 2 2 2
  line L166 (108.5756, 72.8849) -> (109.1245, 72.8849)
  line L167 (110.2393, 71.5777) -> (110.2393, 74.8031)
  line L168 (110.2393, 74.8031) -> (111.1446, 74.8031)
  line L169 (111.1446, 74.8031) -> (111.1446, 71.5777)
  line L170 (111.1446, 71.5777) -> (110.2393, 71.5777)
  spline S142 degree 2 poles (112.3612, 72.4095) (112.3839, 72.2681) (112.6612, 72.1096) (112.8875, 72.1096) knots 0 0 0 1 2 2 2
  spline S143 degree 2 poles (112.8875, 72.1096) (113.2044, 72.1096) (113.4873, 72.2313) knots 0 0 0 1 1 1
  line L171 (113.4873, 72.2313) -> (113.4873, 71.6569)
  spline S144 degree 2 poles (113.4873, 71.6569) (113.1591, 71.524) (112.6866, 71.524) knots 0 0 0 1 1 1
  spline S145 degree 2 poles (112.6866, 71.524) (112.1179, 71.524) (111.4842, 72.1068) (111.4842, 72.6189) knots 0 0 0 1 2 2 2
  spline S146 degree 2 poles (111.4842, 72.6189) (111.4842, 72.9697) (111.7614, 73.5045) (112.3075, 73.81) (112.6385, 73.81) knots 0 0 0 1 2 3 3 3
  spline S147 degree 2 poles (112.6385, 73.81) (112.9752, 73.81) (113.4562, 73.5469) (113.7052, 73.0688) (113.7052, 72.749) knots 0 0 0 1 2 3 3 3
  line L172 (113.7052, 72.749) -> (113.7052, 72.4095)
  line L173 (113.7052, 72.4095) -> (112.3612, 72.4095)
  spline S148 degree 2 poles (112.9045, 72.8849) (112.9045, 73.2612) (112.6357, 73.2612) knots 0 0 0 1 1 1
  spline S149 degree 2 poles (112.6357, 73.2612) (112.5225, 73.2612) (112.3697, 73.0546) (112.3556, 72.8849) knots 0 0 0 1 2 2 2
  line L174 (112.3556, 72.8849) -> (112.9045, 72.8849)
  spline S150 degree 2 poles (69.93, 66.6794) (69.93, 66.5153) (69.7603, 66.2239) (69.4689, 66.057) (69.3076, 66.057) knots 0 0 0 1 2 3 3 3
  spline S151 degree 2 poles (69.3076, 66.057) (69.0558, 66.057) (68.6936, 66.4191) (68.6936, 66.6794) knots 0 0 0 1 2 2 2
  spline S152 degree 2 poles (68.6936, 66.6794) (68.6936, 66.9312) (69.0501, 67.2934) (69.3076, 67.2934) knots 0 0 0 1 2 2 2
  spline S153 degree 2 poles (69.3076, 67.2934) (69.5707, 67.2934) (69.93, 66.9256) (69.93, 66.6794) knots 0 0 0 1 2 2 2
  line L175 (79.7195, 65.641) -> (79.5865, 66.2013)
  line L176 (79.5865, 66.2013) -> (78.6754, 66.2013)
  line L177 (78.6754, 66.2013) -> (78.5311, 65.641)
  line L178 (78.5311, 65.641) -> (77.5381, 65.641)
  line L179 (77.5381, 65.641) -> (78.5877, 68.691)
  line L180 (78.5877, 68.691) -> (79.7279, 68.691)
  line L181 (79.7279, 68.691) -> (80.7182, 65.641)
  line L182 (80.7182, 65.641) -> (79.7195, 65.641)
  line L183 (79.1423, 68.0262) -> (79.1225, 68.0262)
  spline S154 degree 2 poles (79.1225, 68.0262) (79.1168, 67.9752) (79.0659, 67.7404) (78.8339, 66.8548) knots 0 0 0 1 2 2 2
  line L184 (78.8339, 66.8548) -> (79.4167, 66.8548)
  line L185 (79.4167, 66.8548) -> (79.2045, 67.6838)
  spline S155 degree 2 poles (79.2045, 67.6838) (79.1593, 67.8677) (79.1423, 68.0262) knots 0 0 0 1 1 1
  line L186 (82.4045, 65.641) -> (82.4045, 66.8294)
  spline S156 degree 2 poles (82.4045, 66.8294) (82.4045, 67.0331) (82.2828, 67.2085) (82.147, 67.2085) knots 0 0 0 1 2 2 2
  spline S157 degree 2 poles (82.147, 67.2085) (82.031, 67.2085) (81.898, 67.0246) (81.898, 66.8831) knots 0 0 0 1 2 2 2
  line L187 (81.898, 66.8831) -> (81.898, 65.641)
  line L188 (81.898, 65.641) -> (80.9926, 65.641)
  line L189 (80.9926, 65.641) -> (80.9926, 67.8196)
  line L190 (80.9926, 67.8196) -> (81.898, 67.8196)
  line L191 (81.898, 67.8196) -> (81.898, 67.4801)
  line L192 (81.898, 67.4801) -> (81.9065, 67.4801)
  spline S158 degree 2 poles (81.9065, 67.4801) (82.014, 67.6668) (82.3818, 67.8734) (82.5969, 67.8734) knots 0 0 0 1 2 2 2
  spline S159 degree 2 poles (82.5969, 67.8734) (83.3099, 67.8734) (83.3099, 66.9708) knots 0 0 0 1 1 1
  line L193 (83.3099, 66.9708) -> (83.3099, 65.641)
  line L194 (83.3099, 65.641) -> (82.4045, 65.641)
  spline S160 degree 2 poles (86.0826, 65.9438) (86.0826, 65.3157) (85.2932, 64.6168) (84.535, 64.6168) knots 0 0 0 1 2 2 2
  spline S161 degree 2 poles (84.535, 64.6168) (84.3312, 64.6168) (83.9465, 64.6819) (83.8644, 64.7215) knots 0 0 0 1 2 2 2
  line L195 (83.8644, 64.7215) -> (83.8644, 65.4317)
  spline S162 degree 2 poles (83.8644, 65.4317) (84.0002, 65.3468) (84.368, 65.2449) (84.5095, 65.2449) knots 0 0 0 1 2 2 2
  spline S163 degree 2 poles (84.5095, 65.2449) (84.8151, 65.2449) (85.18, 65.5392) (85.18, 65.7825) knots 0 0 0 1 2 2 2
  line L196 (85.18, 65.7825) -> (85.18, 65.9155)
  line L197 (85.18, 65.9155) -> (85.1715, 65.9155)
  spline S164 degree 2 poles (85.1715, 65.9155) (85.0725, 65.7655) (84.7302, 65.5873) (84.535, 65.5873) knots 0 0 0 1 2 2 2
  spline S165 degree 2 poles (84.535, 65.5873) (84.1134, 65.5873) (83.6239, 66.173) (83.6239, 66.6879) knots 0 0 0 1 2 2 2
  spline S166 degree 2 poles (83.6239, 66.6879) (83.6239, 67.0416) (83.8785, 67.582) (84.3341, 67.8734) (84.6085, 67.8734) knots 0 0 0 1 2 3 3 3
  spline S167 degree 2 poles (84.6085, 67.8734) (84.9876, 67.8734) (85.1715, 67.5933) knots 0 0 0 1 1 1
  line L198 (85.1715, 67.5933) -> (85.18, 67.5933)
  line L199 (85.18, 67.5933) -> (85.18, 67.8196)
  line L200 (85.18, 67.8196) -> (86.0826, 67.8196)
  line L201 (86.0826, 67.8196) -> (86.0826, 65.9438)
  spline S168 degree 2 poles (85.1942, 66.7926) (85.1942, 66.9821) (85.0216, 67.2085) (84.8801, 67.2085) knots 0 0 0 1 2 2 2
  spline S169 degree 2 poles (84.8801, 67.2085) (84.7273, 67.2085) (84.5434, 66.9369) (84.5434, 66.7077) knots 0 0 0 1 2 2 2
  spline S170 degree 2 poles (84.5434, 66.7077) (84.5434, 66.4983) (84.6962, 66.2522) (84.8632, 66.2522) knots 0 0 0 1 2 2 2
  spline S171 degree 2 poles (84.8632, 66.2522) (85.0188, 66.2522) (85.1942, 66.504) (85.1942, 66.719) knots 0 0 0 1 2 2 2
  line L202 (85.1942, 66.719) -> (85.1942, 66.7926)
  spline S172 degree 2 poles (87.2992, 66.4729) (87.3218, 66.3314) (87.5991, 66.173) (87.8254, 66.173) knots 0 0 0 1 2 2 2
  spline S173 degree 2 poles (87.8254, 66.173) (88.1423, 66.173) (88.4253, 66.2946) knots 0 0 0 1 1 1
  line L203 (88.4253, 66.2946) -> (88.4253, 65.7203)
  spline S174 degree 2 poles (88.4253, 65.7203) (88.0971, 65.5873) (87.6246, 65.5873) knots 0 0 0 1 1 1
  spline S175 degree 2 poles (87.6246, 65.5873) (87.0559, 65.5873) (86.4221, 66.1701) (86.4221, 66.6822) knots 0 0 0 1 2 2 2
  spline S176 degree 2 poles (86.4221, 66.6822) (86.4221, 67.0331) (86.6994, 67.5678) (87.2454, 67.8734) (87.5765, 67.8734) knots 0 0 0 1 2 3 3 3
  spline S177 degree 2 poles (87.5765, 67.8734) (87.9132, 67.8734) (88.3941, 67.6103) (88.6431, 67.1321) (88.6431, 66.8124) knots 0 0 0 1 2 3 3 3
  line L204 (88.6431, 66.8124) -> (88.6431, 66.4729)
  line L205 (88.6431, 66.4729) -> (87.2992, 66.4729)
  spline S178 degree 2 poles (87.8424, 66.9482) (87.8424, 67.3245) (87.5736, 67.3245) knots 0 0 0 1 1 1
  spline S179 degree 2 poles (87.5736, 67.3245) (87.4605, 67.3245) (87.3077, 67.118) (87.2935, 66.9482) knots 0 0 0 1 2 2 2
  line L206 (87.2935, 66.9482) -> (87.8424, 66.9482)
  line L207 (88.9572, 65.641) -> (88.9572, 68.8665)
  line L208 (88.9572, 68.8665) -> (89.8625, 68.8665)
  line L209 (89.8625, 68.8665) -> (89.8625, 65.641)
  line L210 (89.8625, 65.641) -> (88.9572, 65.641)
  spline S180 degree 2 poles (92.7202, 66.7699) (92.7202, 66.2182) (92.0553, 65.5873) (91.4583, 65.5873) knots 0 0 0 1 2 2 2
  spline S181 degree 2 poles (91.4583, 65.5873) (90.8641, 65.5873) (90.2021, 66.2013) (90.2021, 66.7445) knots 0 0 0 1 2 2 2
  spline S182 degree 2 poles (90.2021, 66.7445) (90.2021, 67.0897) (90.5133, 67.6018) (91.0876, 67.8734) (91.4611, 67.8734) knots 0 0 0 1 2 3 3 3
  spline S183 degree 2 poles (91.4611, 67.8734) (91.8487, 67.8734) (92.4174, 67.5876) (92.7202, 67.0812) (92.7202, 66.7699) knots 0 0 0 1 2 3 3 3
  spline S184 degree 2 poles (91.8006, 66.7643) (91.8006, 67.2085) (91.4611, 67.2085) knots 0 0 0 1 1 1
  spline S185 degree 2 poles (91.4611, 67.2085) (91.1216, 67.2085) (91.1216, 66.7445) knots 0 0 0 1 1 1
  spline S186 degree 2 poles (91.1216, 66.7445) (91.1216, 66.2522) (91.4668, 66.2522) knots 0 0 0 1 1 1
  spline S187 degree 2 poles (91.4668, 66.2522) (91.8006, 66.2522) (91.8006, 66.7643) knots 0 0 0 1 1 1
  line L211 (94.4715, 65.641) -> (94.4715, 66.8294)
  spline S188 degree 2 poles (94.4715, 66.8294) (94.4715, 67.0331) (94.3498, 67.2085) (94.214, 67.2085) knots 0 0 0 1 2 2 2
  spline S189 degree 2 poles (94.214, 67.2085) (94.098, 67.2085) (93.9651, 67.0246) (93.9651, 66.8831) knots 0 0 0 1 2 2 2
  line L212 (93.9651, 66.8831) -> (93.9651, 65.641)
  line L213 (93.9651, 65.641) -> (93.0597, 65.641)
  line L214 (93.0597, 65.641) -> (93.0597, 67.8196)
  line L215 (93.0597, 67.8196) -> (93.9651, 67.8196)
  line L216 (93.9651, 67.8196) -> (93.9651, 67.4801)
  line L217 (93.9651, 67.4801) -> (93.9735, 67.4801)
  spline S190 degree 2 poles (93.9735, 67.4801) (94.0811, 67.6668) (94.4489, 67.8734) (94.6639, 67.8734) knots 0 0 0 1 2 2 2
  spline S191 degree 2 poles (94.6639, 67.8734) (95.3769, 67.8734) (95.3769, 66.9708) knots 0 0 0 1 1 1
  line L218 (95.3769, 66.9708) -> (95.3769, 65.641)
  line L219 (95.3769, 65.641) -> (94.4715, 65.641)
  line L220 (95.7871, 65.641) -> (95.7871, 67.8196)
  line L221 (95.7871, 67.8196) -> (96.6925, 67.8196)
  line L222 (96.6925, 67.8196) -> (96.6925, 65.641)
  line L223 (96.6925, 65.641) -> (95.7871, 65.641)
  spline S192 degree 2 poles (96.7463, 68.4081) (96.7463, 68.2157) (96.4662, 67.9781) (96.2398, 67.9781) knots 0 0 0 1 2 2 2
  spline S193 degree 2 poles (96.2398, 67.9781) (96.0191, 67.9781) (95.7362, 68.2242) (95.7362, 68.4081) knots 0 0 0 1 2 2 2
  spline S194 degree 2 poles (95.7362, 68.4081) (95.7362, 68.5949) (96.0106, 68.8269) (96.2398, 68.8269) knots 0 0 0 1 2 2 2
  spline S195 degree 2 poles (96.2398, 68.8269) (96.4662, 68.8269) (96.7463, 68.5949) (96.7463, 68.4081) knots 0 0 0 1 2 2 2
  line L224 (98.4212, 65.641) -> (98.4212, 68.691)
  line L225 (98.4212, 68.691) -> (99.3407, 68.691)
  line L226 (99.3407, 68.691) -> (99.3407, 65.641)
  line L227 (99.3407, 65.641) -> (98.4212, 65.641)
  line L228 (99.8585, 65.641) -> (99.8585, 68.8665)
  line L229 (99.8585, 68.8665) -> (100.7639, 68.8665)
  line L230 (100.7639, 68.8665) -> (100.7639, 65.641)
  line L231 (100.7639, 65.641) -> (99.8585, 65.641)
  line L232 (102.4077, 65.641) -> (102.4077, 65.9721)
  line L233 (102.4077, 65.9721) -> (102.3992, 65.9721)
  spline S196 degree 2 poles (102.3992, 65.9721) (102.1814, 65.5873) (101.7343, 65.5873) knots 0 0 0 1 1 1
  spline S197 degree 2 poles (101.7343, 65.5873) (101.426, 65.5873) (101.0779, 65.9523) (101.0779, 66.2607) knots 0 0 0 1 2 2 2
  spline S198 degree 2 poles (101.0779, 66.2607) (101.0779, 66.9029) (101.8673, 67.0048) knots 0 0 0 1 1 1
  line L234 (101.8673, 67.0048) -> (102.4077, 67.0755)
  spline S199 degree 2 poles (102.4077, 67.0755) (102.4077, 67.183) (102.2153, 67.3188) (102.0541, 67.3188) knots 0 0 0 1 2 2 2
  spline S200 degree 2 poles (102.0541, 67.3188) (101.6891, 67.3188) (101.2817, 67.1095) knots 0 0 0 1 1 1
  line L235 (101.2817, 67.1095) -> (101.2817, 67.698)
  spline S201 degree 2 poles (101.2817, 67.698) (101.4571, 67.7744) (101.9918, 67.8734) (102.1814, 67.8734) knots 0 0 0 1 2 2 2
  spline S202 degree 2 poles (102.1814, 67.8734) (102.7359, 67.8734) (103.2367, 67.3981) (103.2367, 66.8435) knots 0 0 0 1 2 2 2
  line L236 (103.2367, 66.8435) -> (103.2367, 65.641)
  line L237 (103.2367, 65.641) -> (102.4077, 65.641)
  spline S203 degree 2 poles (101.8702, 66.3823) (101.8702, 66.2946) (101.9833, 66.1786) (102.088, 66.1786) knots 0 0 0 1 2 2 2
  spline S204 degree 2 poles (102.088, 66.1786) (102.2295, 66.1786) (102.4077, 66.3908) (102.4077, 66.5577) knots 0 0 0 1 2 2 2
  line L238 (102.4077, 66.5577) -> (102.4077, 66.6398)
  line L239 (102.4077, 66.6398) -> (102.0993, 66.5974)
  spline S205 degree 2 poles (102.0993, 66.5974) (101.8702, 66.5577) (101.8702, 66.3823) knots 0 0 0 1 1 1
  spline S206 degree 2 poles (105.2823, 67.0444) (105.2314, 67.067) (105.056, 67.1038) (104.9994, 67.1038) knots 0 0 0 1 2 2 2
  spline S207 degree 2 poles (104.9994, 67.1038) (104.5495, 67.1038) (104.5495, 66.586) knots 0 0 0 1 1 1
  line L240 (104.5495, 66.586) -> (104.5495, 65.641)
  line L241 (104.5495, 65.641) -> (103.6441, 65.641)
  line L242 (103.6441, 65.641) -> (103.6441, 67.8196)
  line L243 (103.6441, 67.8196) -> (104.5495, 67.8196)
  line L244 (104.5495, 67.8196) -> (104.5495, 67.4377)
  line L245 (104.5495, 67.4377) -> (104.558, 67.4377)
  spline S208 degree 2 poles (104.558, 67.4377) (104.6401, 67.6442) (104.9484, 67.8592) (105.1522, 67.8592) knots 0 0 0 1 2 2 2
  spline S209 degree 2 poles (105.1522, 67.8592) (105.2257, 67.8592) (105.2823, 67.8338) knots 0 0 0 1 1 1
  line L246 (105.2823, 67.8338) -> (105.2823, 67.0444)
  line L247 (105.5426, 65.641) -> (105.5426, 67.8196)
  line L248 (105.5426, 67.8196) -> (106.448, 67.8196)
  line L249 (106.448, 67.8196) -> (106.448, 65.641)
  line L250 (106.448, 65.641) -> (105.5426, 65.641)
  spline S210 degree 2 poles (106.5017, 68.4081) (106.5017, 68.2157) (106.2216, 67.9781) (105.9953, 67.9781) knots 0 0 0 1 2 2 2
  spline S211 degree 2 poles (105.9953, 67.9781) (105.7746, 67.9781) (105.4917, 68.2242) (105.4917, 68.4081) knots 0 0 0 1 2 2 2
  spline S212 degree 2 poles (105.4917, 68.4081) (105.4917, 68.5949) (105.7661, 68.8269) (105.9953, 68.8269) knots 0 0 0 1 2 2 2
  spline S213 degree 2 poles (105.9953, 68.8269) (106.2216, 68.8269) (106.5017, 68.5949) (106.5017, 68.4081) knots 0 0 0 1 2 2 2
  line L251 (108.0918, 65.641) -> (108.0918, 65.9721)
  line L252 (108.0918, 65.9721) -> (108.0833, 65.9721)
  spline S214 degree 2 poles (108.0833, 65.9721) (107.8655, 65.5873) (107.4184, 65.5873) knots 0 0 0 1 1 1
  spline S215 degree 2 poles (107.4184, 65.5873) (107.11, 65.5873) (106.762, 65.9523) (106.762, 66.2607) knots 0 0 0 1 2 2 2
  spline S216 degree 2 poles (106.762, 66.2607) (106.762, 66.9029) (107.5514, 67.0048) knots 0 0 0 1 1 1
  line L253 (107.5514, 67.0048) -> (108.0918, 67.0755)
  spline S217 degree 2 poles (108.0918, 67.0755) (108.0918, 67.183) (107.8994, 67.3188) (107.7382, 67.3188) knots 0 0 0 1 2 2 2
  spline S218 degree 2 poles (107.7382, 67.3188) (107.3732, 67.3188) (106.9657, 67.1095) knots 0 0 0 1 1 1
  line L254 (106.9657, 67.1095) -> (106.9657, 67.698)
  spline S219 degree 2 poles (106.9657, 67.698) (107.1412, 67.7744) (107.6759, 67.8734) (107.8655, 67.8734) knots 0 0 0 1 2 2 2
  spline S220 degree 2 poles (107.8655, 67.8734) (108.42, 67.8734) (108.9208, 67.3981) (108.9208, 66.8435) knots 0 0 0 1 2 2 2
  line L255 (108.9208, 66.8435) -> (108.9208, 65.641)
  line L256 (108.9208, 65.641) -> (108.0918, 65.641)
  spline S221 degree 2 poles (107.5542, 66.3823) (107.5542, 66.2946) (107.6674, 66.1786) (107.7721, 66.1786) knots 0 0 0 1 2 2 2
  spline S222 degree 2 poles (107.7721, 66.1786) (107.9136, 66.1786) (108.0918, 66.3908) (108.0918, 66.5577) knots 0 0 0 1 2 2 2
  line L257 (108.0918, 66.5577) -> (108.0918, 66.6398)
  line L258 (108.0918, 66.6398) -> (107.7834, 66.5974)
  spline S223 degree 2 poles (107.7834, 66.5974) (107.5542, 66.5577) (107.5542, 66.3823) knots 0 0 0 1 1 1
  spline S224 degree 2 poles (69.93, 60.7427) (69.93, 60.5786) (69.7603, 60.2872) (69.4689, 60.1203) (69.3076, 60.1203) knots 0 0 0 1 2 3 3 3
  spline S225 degree 2 poles (69.3076, 60.1203) (69.0558, 60.1203) (68.6936, 60.4824) (68.6936, 60.7427) knots 0 0 0 1 2 2 2
  spline S226 degree 2 poles (68.6936, 60.7427) (68.6936, 60.9946) (69.0501, 61.3567) (69.3076, 61.3567) knots 0 0 0 1 2 2 2
  spline S227 degree 2 poles (69.3076, 61.3567) (69.5707, 61.3567) (69.93, 60.9889) (69.93, 60.7427) knots 0 0 0 1 2 2 2
  line L259 (79.7195, 59.7044) -> (79.5865, 60.2646)
  line L260 (79.5865, 60.2646) -> (78.6754, 60.2646)
  line L261 (78.6754, 60.2646) -> (78.5311, 59.7044)
  line L262 (78.5311, 59.7044) -> (77.5381, 59.7044)
  line L263 (77.5381, 59.7044) -> (78.5877, 62.7544)
  line L264 (78.5877, 62.7544) -> (79.7279, 62.7544)
  line L265 (79.7279, 62.7544) -> (80.7182, 59.7044)
  line L266 (80.7182, 59.7044) -> (79.7195, 59.7044)
  line L267 (79.1423, 62.0895) -> (79.1225, 62.0895)
  spline S228 degree 2 poles (79.1225, 62.0895) (79.1168, 62.0386) (79.0659, 61.8037) (78.8339, 60.9182) knots 0 0 0 1 2 2 2
  line L268 (78.8339, 60.9182) -> (79.4167, 60.9182)
  line L269 (79.4167, 60.9182) -> (79.2045, 61.7471)
  spline S229 degree 2 poles (79.2045, 61.7471) (79.1593, 61.9311) (79.1423, 62.0895) knots 0 0 0 1 1 1
  line L270 (82.4045, 59.7044) -> (82.4045, 60.8927)
  spline S230 degree 2 poles (82.4045, 60.8927) (82.4045, 61.0964) (82.2828, 61.2718) (82.147, 61.2718) knots 0 0 0 1 2 2 2
  spline S231 degree 2 poles (82.147, 61.2718) (82.031, 61.2718) (81.898, 61.0879) (81.898, 60.9465) knots 0 0 0 1 2 2 2
  line L271 (81.898, 60.9465) -> (81.898, 59.7044)
  line L272 (81.898, 59.7044) -> (80.9926, 59.7044)
  line L273 (80.9926, 59.7044) -> (80.9926, 61.883)
  line L274 (80.9926, 61.883) -> (81.898, 61.883)
  line L275 (81.898, 61.883) -> (81.898, 61.5434)
  line L276 (81.898, 61.5434) -> (81.9065, 61.5434)
  spline S232 degree 2 poles (81.9065, 61.5434) (82.014, 61.7302) (82.3818, 61.9367) (82.5969, 61.9367) knots 0 0 0 1 2 2 2
  spline S233 degree 2 poles (82.5969, 61.9367) (83.3099, 61.9367) (83.3099, 61.0342) knots 0 0 0 1 1 1
  line L277 (83.3099, 61.0342) -> (83.3099, 59.7044)
  line L278 (83.3099, 59.7044) -> (82.4045, 59.7044)
  spline S234 degree 2 poles (85.2536, 59.7327) (85.1914, 59.7044) (84.9112, 59.6506) (84.7132, 59.6506) knots 0 0 0 1 2 2 2
  spline S235 degree 2 poles (84.7132, 59.6506) (84.3341, 59.6506) (83.9068, 60.0665) (83.9068, 60.4542) knots 0 0 0 1 2 2 2
  line L279 (83.9068, 60.4542) -> (83.9068, 61.2548)
  line L280 (83.9068, 61.2548) -> (83.5645, 61.2548)
  line L281 (83.5645, 61.2548) -> (83.5645, 61.883)
  line L282 (83.5645, 61.883) -> (83.9068, 61.883)
  line L283 (83.9068, 61.883) -> (83.9068, 62.3102)
  line L284 (83.9068, 62.3102) -> (84.8009, 62.5563)
  line L285 (84.8009, 62.5563) -> (84.8009, 61.883)
  line L286 (84.8009, 61.883) -> (85.2536, 61.883)
  line L287 (85.2536, 61.883) -> (85.2536, 61.2548)
  line L288 (85.2536, 61.2548) -> (84.8009, 61.2548)
  line L289 (84.8009, 61.2548) -> (84.8009, 60.6013)
  spline S236 degree 2 poles (84.8009, 60.6013) (84.8009, 60.3155) (85.0273, 60.3155) knots 0 0 0 1 1 1
  spline S237 degree 2 poles (85.0273, 60.3155) (85.1348, 60.3155) (85.2536, 60.3608) knots 0 0 0 1 1 1
  line L290 (85.2536, 60.3608) -> (85.2536, 59.7327)
  spline S238 degree 2 poles (87.9584, 60.8333) (87.9584, 60.2816) (87.2935, 59.6506) (86.6965, 59.6506) knots 0 0 0 1 2 2 2
  spline S239 degree 2 poles (86.6965, 59.6506) (86.1024, 59.6506) (85.4403, 60.2646) (85.4403, 60.8078) knots 0 0 0 1 2 2 2